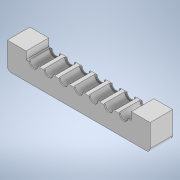
# Autodesk Inventor part: top_bot_insert
Saved by Autodesk Inventor 2021 (Build 250183000, 183)
## iProperties
Created: 2021-06-03
Part Number: top_bot_insert
Material: Generic
Document SubType Name: Modeling
Designer: Anton
Density: 1 g/cm^3
Appearance: Default
Author: Anton
Autodesk Inventor part; units mm, degrees
ref_plane "YZ Plane" through (0, 0, 0) normal (1, 0, 0) x (0, 1, 0)
ref_plane "XZ Plane" through (0, 0, 0) normal (0, 1, 0) x (-1, 0, 0)
ref_plane "XY Plane" through (0, 0, 0) normal (0, 0, 1) x (1, 0, 0)
sketch "Sketch1" plane through (0, 0, 0) normal (0, 0, 1) x (1, 0, 0)
  line L0 (0, 0) -> (76, 0)
  line L1 (76, 0) -> (76, 28)
  line L2 (76, 28) -> (0, 28)
  line L3 (0, 28) -> (0, 0)
  line L4 (10, 18) -> (66, 18)
  line L5 (66, 18) -> (66, 10)
  line L6 (66, 10) -> (10, 10)
  line L7 (10, 10) -> (10, 18)
  circle A0 centre (14, 18) radius 3
  circle A1 centre (14, 10) radius 3
  circle A2 centre (22, 18) radius 3
  circle A3 centre (22, 10) radius 3
  circle A4 centre (30, 18) radius 3
  circle A5 centre (30, 10) radius 3
  circle A6 centre (38, 18) radius 3
  circle A7 centre (38, 10) radius 3
  circle A8 centre (46, 18) radius 3
  circle A9 centre (46, 10) radius 3
  circle A10 centre (54, 18) radius 3
  circle A11 centre (54, 10) radius 3
  circle A12 centre (62, 18) radius 3
  circle A13 centre (62, 10) radius 3
  line L8 (10, 14) -> (0, 14)
  line L9 (66, 14) -> (76, 14)
  point P0 (65, 10)
  point P1 (59, 10)
  point P2 (57, 10)
  point P3 (51, 10)
  point P4 (49, 10)
  point P5 (43, 10)
  point P6 (41, 10)
  point P7 (35, 10)
  point P8 (33, 10)
  point P9 (27, 10)
  point P10 (25, 10)
  point P11 (19, 10)
  point P12 (17, 10)
  point P13 (11, 10)
  dimension "d2" = 56
  dimension "d3" = 8
  dimension "d4" = 10
  dimension "d5" = 10
  dimension "d6" = 10
  dimension "d7" = 10
  dimension "d8" = 6
  dimension "d9" = 6
  dimension "d10" = 4
  dimension "d11" = 4
  dimension "d14" = 8
  constraints: 20 end point, 14 centre point, 4 midpoint, 4 parallel, 3 horizontal, 2 perpendicular, 2 point on line, 24 other
  measures "d2" distance between parallel lines of L5 L7
  measures "d3" distance between parallel lines of L6 L4
  measures "d4" distance between parallel lines of L2 L4
  measures "d5" distance between parallel lines of L0 L6
  measures "d6" distance between parallel lines of L5 L1
  measures "d7" distance between parallel lines of L3 L7
  measures "d8" diameter of A0
  measures "d9" diameter of A1
  measures "d10" distance from line of L7 A0.centre
  measures "d11" distance from line of L7 A1.centre
  measures "d14" distance of A0.centre A2.centre
extrude "Extrusion1" add sketch "Sketch1" along normal blind 11 contours L3 L8 L7 L6 A1 A3 A5 A7 A9 A11 A13 L5 L9 L1 L0
sketch "Sketch2" plane through (0, 0, 0) normal (0, 0, -1) x (-1, 0, 0)
  line L0 (0, 0) -> (-76, 0) projected
  line L1 (-76, 0) -> (-76, 14) projected
  line L2 (0, 0) -> (-76, 0)
  line L3 (-76, 0) -> (-76, 14)
  line L4 (-76, 14) -> (0, 14)
  line L5 (0, 14) -> (0, 0)
  constraints: 8 end point, 2 parallel, 1 horizontal, 1 perpendicular
extrude "Extrusion2" add sketch "Sketch2" along normal blind 0.5
sketch "Sketch3" plane through (0, 0, 11) normal (0, 0, 1) x (1, 0, 0)
  line L0 (76, 14) -> (66, 14) projected
  line L1 (0, 0) -> (76, 0)
  line L2 (76, 0) -> (76, 14)
  line L3 (76, 14) -> (0, 14)
  line L4 (0, 14) -> (0, 0)
  constraints: 8 end point, 2 parallel, 1 horizontal, 1 perpendicular
extrude "Extrusion3" add sketch "Sketch3" along normal blind 0.5
sketch "Sketch4" plane through (0, 0, -0.5) normal (0, 0, -1) x (-1, 0, 0)
  line L0 (0, 14) -> (-76, 14) projected
  line L1 (-66, 14) -> (-10, 14)
  line L2 (-10, 14) -> (-10, 10)
  line L3 (-10, 10) -> (-66, 10)
  line L4 (-66, 10) -> (-66, 14)
  point P0 (0, 0)
  dimension "d27" = 4
  dimension "d28" = 56
  constraints: 8 end point, 2 parallel, 1 horizontal, 1 perpendicular
  measures "d27" distance between parallel lines of L0 L3
  measures "d28" distance between parallel lines of L2 L4
extrude "Extrusion4" cut sketch "Sketch4" along normal mid plane 100
sketch "Sketch5" plane through (0, 0, -0.5) normal (0, 0, -1) x (-1, 0, 0)
  line L0 (-65, 10) -> (-59, 10) projected
  circle A0 centre (-62, 10) radius 2.25
  circle A1 centre (-54, 10) radius 2.25
  circle A2 centre (-46, 10) radius 2.25
  circle A3 centre (-38, 10) radius 2.25
  circle A4 centre (-30, 10) radius 2.25
  circle A5 centre (-22, 10) radius 2.25
  circle A6 centre (-14, 10) radius 2.25
  point P0 (0, 0)
  point P1 (-59.75, 10)
  point P2 (-64.25, 10)
  dimension "d31" = 4.5
  dimension "d34" = 8
  constraints: 7 centre point, 1 horizontal, 1 midpoint, 12 other
  measures "d31" diameter of A0
  measures "d34" distance of A0.centre A1.centre
extrude "Extrusion5" cut sketch "Sketch5" along normal mid plane 100 contours L0 A0 | A1 | A2 | A3 | A4 | A5 | A6 picked at (-61.488, 9.0342)
fillet "Fillet1" radius 2 2 edges at (76, 0, 5.5) (0, 0, 5.5)
body "Solid1"
